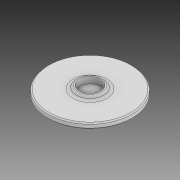
# Autodesk Inventor part: ElectromagnetEnds
Saved by Autodesk Inventor 2020 (Build 240168000, 168)
## iProperties
Created: 2021-03-10
Part Number: ElectromagnetEnds
Material: Generic
Document SubType Name: Modeling
Designer: DDeGo
Density: 1 g/cm^3
Appearance: Default
Author: DDeGo
Autodesk Inventor part; units mm, degrees
ref_plane "YZ Plane" through (0, 0, 0) normal (1, 0, 0) x (0, 1, 0)
ref_plane "XZ Plane" through (0, 0, 0) normal (0, 1, 0) x (-1, 0, 0)
ref_plane "XY Plane" through (0, 0, 0) normal (0, 0, 1) x (1, 0, 0)
sketch "Sketch1" plane through (0, 0, 0) normal (1, 0, 0) x (0, 1, 0)
  line L0 (0, 0) -> (0, -7)
  line L1 (0.5, -19) -> (2, -19)
  line L2 (2.5, -18.5) -> (2.5, -7.6284)
  line L3 (2.5, -4.8) -> (1, -4.8)
  line L4 (1, -4.8) -> (1, 0)
  line L5 (1, 0) -> (0, 0)
  line L6 (0.5, -19) -> (0, -18.5)
  line L7 (0, -7) -> (1.5, -7.25)
  line L8 (1.5, -7.25) -> (1.5, -8.75)
  line L9 (1.5, -8.75) -> (0, -9)
  line L10 (0, -7) -> (0, -9) construction
  line L11 (0, -9) -> (0, -18.5)
  line L12 (2.5, -4.8) -> (4, -4.8)
  line L13 (4, -4.8) -> (4, -5.3)
  line L14 (4, -5.3) -> (3.0858, -6.2142)
  line L15 (2.5, -6.8) -> (2.5, -4.8) construction
  arc A0 (3.0858, -6.2142) -> (2.5, -7.6284) centre (4.5, -7.6284) ccw
  line L16 (2.5, -18.5) -> (2, -19)
  point P0 (0, -19)
  point P1 (2.5, -19)
  point P2 (0, -8)
  dimension "d0" = 4.8
  dimension "d1" = 1.5
  dimension "d2" = 1
  dimension "d3" = 19
  dimension "d5" = 0.5
  dimension "d6" = 0.5
  dimension "d7" = 1.5
  dimension "d8" = 1.5
  dimension "d9" = 2
  dimension "d10" = 8
  dimension "d19" = 135
  dimension "d20" = 1.5
  dimension "d21" = 0.5
  dimension "d22" = 2
  dimension "d23" = 0.5
  dimension "d24" = 0.5
  constraints: 34 end point, 10 perpendicular, 7 point on line, 4 vertical, 2 point on circle, 2 tangent, 1 centre point, 1 equal length, 1 horizontal, 1 midpoint
  measures "d0" distance between parallel lines of L3 L5
  measures "d1" distance of L3.start L3.end
  measures "d2" distance between parallel lines of L0 L4
  measures "d3" distance between parallel lines of L5 L1
  measures "d5" distance of L1.start point (0, -19)
  measures "d6" distance of L6.end point (0, -19)
  measures "d7" distance between parallel lines of L10 L8
  measures "d8" distance of L7.end L8.end
  measures "d9" distance of L0.end L9.end
  measures "d10" distance from line of L5 point (0, -8)
  measures "d19" angle of L13 L14
  measures "d20" distance of L3.start L12.end
  measures "d21" distance of L12.end L13.end
  measures "d22" radius of A0
  measures "d23" distance of L2.start point (2.5, -19)
  measures "d24" distance of L1.end point (2.5, -19)
revolve "Revolution1" add sketch "Sketch1" angle 360 about axis through (0, 1, 0) along (0, -1, 0)
sketch "Sketch2" plane through (0, 0, 0) normal (0, -1, 0) x (1, 0, 0)
  line L0 (0, 0) -> (13, 0) construction
  circle A0 centre (13, 0) radius 2
  dimension "d11" = 13
  dimension "d12" = 4
  constraints: 2 end point, 1 centre point, 1 coincident, 1 horizontal
  measures "d11" distance of L0.start L0.end
  measures "d12" diameter of A0
extrude "Extrusion1" cut sketch "Sketch2" against normal blind 1.6
fillet "Fillet1" radius 0.8 1 edges at (11, 0, 0)
pattern_circular "Circular Pattern1" count 12 over 360 about axis through (0, 1.25, 0) along (0, -1, 0) of "Extrusion1", "Fillet1"
equation "\"d6\" = d5"
equation "\"d23\" = d5"
equation "\"d24\" = d23"
body "Solid1"
